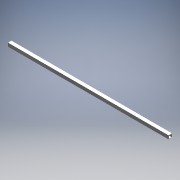
# Autodesk Inventor part: Main Extrusions
Saved by Autodesk Inventor 2019.4 (Build 234330000, 330)
## iProperties
Created: 2020-01-18
Part Number: Main Extrusions
Material: Aluminum 6061
Document SubType Name: Modeling
Designer: Mark
Mass: 349.92 g
Surface Area: 1301.99 cm^2
Volume: 129.6 cm^3
Density: 2.7 g/cm^3
Appearance: Aluminum - Flat
Author: Mark
Autodesk Inventor part; units mm, degrees
ref_plane "YZ Plane" through (0, 0, 0) normal (1, 0, 0) x (0, 1, 0)
ref_plane "XZ Plane" through (0, 0, 0) normal (0, 1, 0) x (-1, 0, 0)
ref_plane "XY Plane" through (0, 0, 0) normal (0, 0, 1) x (1, 0, 0)
sketch "Sketch1" plane through (0, 0, 0) normal (1, 0, 0) x (0, 1, 0)
  line L0 (-10, 10) -> (10, 10)
  line L1 (10, 10) -> (10, -10)
  line L2 (10, -10) -> (-10, -10)
  line L3 (-10, -10) -> (-10, 10)
  line L4 (-10, 10) -> (10, -10) construction
  line L5 (10, 10) -> (-10, -10) construction
  line L6 (-8, 8) -> (8, 8)
  line L7 (8, 8) -> (8, -8)
  line L8 (8, -8) -> (-8, -8)
  line L9 (-8, -8) -> (-8, 8)
  line L10 (-8, 8) -> (8, -8) construction
  line L11 (8, 8) -> (-8, -8) construction
  point P0 (0, 0)
  dimension "d0" = 20
  dimension "d1" = 20
  dimension "d2" = 16
  dimension "d3" = 16
  constraints: 24 end point, 4 midpoint, 4 parallel, 2 horizontal, 2 perpendicular
  measures "d0" distance of L1.end L2.end
  measures "d1" distance of L0.end L1.end
  measures "d2" distance of L7.end L8.end
  measures "d3" distance of L6.end L7.end
extrude "Extrusion1" add sketch "Sketch1" along normal blind 930
sketch "Sketch2" plane through (0, -10, -10) normal (0, 0, -1) x (-1, 0, 0)
  line L0 (-930, 0) -> (-930, 20) projected
  line L1 (-930, 0) -> (-870, 20)
  line L2 (0, 20) -> (-930, 20) projected
  point P0 (0, 10)
  dimension "d6" = 60
  constraints: 2 end point, 1 point on line
  measures "d6" distance from line of L0 L1.end
extrude "Extrusion2" cut sketch "Sketch2" against normal blind 20
body "Solid1"
